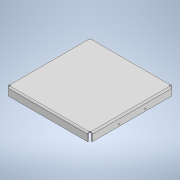
# Autodesk Inventor part: sheetmetaltop2.0
Saved by Autodesk Inventor 2020.2 (Build 242310000, 310)
## iProperties
Created: 2020-02-06
Part Number: sheetmetaltop2.0
Material: Generic
Document SubType Name: Sheet Metal
Designer: ColinP
Density: 1 g/cm^3
Sheet Metal Rule: Default
Appearance: Default
Flat Pattern Width: 27.94 cm
Flat Pattern Length: 27.94 cm
Flat Pattern Area: 780.644 cm^2
Sheet Metal Width: 11.000 in
Sheet Metal Length: 11.000 in
Sheet Metal Area: 121.000 in^2
Author: ColinP
Autodesk Inventor part; units mm, degrees
ref_plane "YZ Plane" through (0, 0, 0) normal (1, 0, 0) x (0, 1, 0)
ref_plane "XZ Plane" through (0, 0, 0) normal (0, 1, 0) x (-1, 0, 0)
ref_plane "XY Plane" through (0, 0, 0) normal (0, 0, 1) x (1, 0, 0)
sketch "Sketch1" plane through (0, 0, 0) normal (0, 1, 0) x (-1, 0, 0)
  line L0 (114.3, 114.3) -> (-114.3, 114.3)
  line L1 (-114.3, 114.3) -> (-114.3, -114.3)
  line L2 (-114.3, -114.3) -> (114.3, -114.3)
  line L3 (114.3, -114.3) -> (114.3, 114.3)
  line L4 (114.3, 114.3) -> (139.7, 114.3)
  line L5 (139.7, 114.3) -> (139.7, -114.3)
  line L6 (139.7, -114.3) -> (114.3, -114.3)
  line L7 (114.3, -114.3) -> (114.3, -139.7)
  line L8 (114.3, -139.7) -> (-114.3, -139.7)
  line L9 (-114.3, -139.7) -> (-114.3, -114.3)
  line L10 (-114.3, -114.3) -> (-139.7, -114.3)
  line L11 (-139.7, -114.3) -> (-139.7, 114.3)
  line L12 (-139.7, 114.3) -> (-114.3, 114.3)
  line L13 (-114.3, 114.3) -> (-114.3, 139.7)
  line L14 (-114.3, 139.7) -> (114.3, 139.7)
  line L15 (114.3, 139.7) -> (114.3, 114.3)
  point P0 (0, 0)
  dimension "d0" = 228.6
  dimension "d1" = 228.6
  dimension "d2" = 25.4
  dimension "d3" = 25.4
  dimension "d4" = 25.4
  dimension "d5" = 25.4
  measures "d0" distance of L2.end L1.end
  measures "d1" distance of L1.end L0.end
  measures "d2" distance of L0.start L4.end
  measures "d3" distance of L2.end L7.end
  measures "d4" distance of L1.end L10.end
  measures "d5" distance of L0.end L13.end
extrude "Plate1" add sketch "Sketch1" along normal blind 3.048
sketch "Sketch3" plane through (0, 0, 0) normal (0, -1, 0) x (1, 0, 0)
  line L0 (-114.3, -114.3) -> (-114.3, -139.7) projected
  line L1 (-114.3, -114.3) -> (-114.3, -116.84)
  line L2 (-114.3, -116.84) -> (114.3, -116.84)
  line L3 (114.3, -139.7) -> (114.3, -114.3) projected
  line L4 (114.3, -116.84) -> (114.3, -114.3)
  point P0 (0, 0)
  dimension "d8" = 2.54
  dimension "d9" = 90
  constraints: 6 end point, 2 point on line
  measures "d8" distance of L0.start L1.end
  measures "d9" angle of L2 L1
fold "Fold1" angle 90 bend radius 1.27 thickness 3.048 k factor 0.44 line from (-114.3, 0, -116.84) to (114.3, 0, -116.84) line at bend start moving side (0, 0, -1) folds toward (0, -1, 0)
sketch "Sketch4" plane through (0, 0, 0) normal (0, -1, 0) x (1, 0, 0)
  line L0 (-139.7, -114.3) -> (-114.3, -114.3) projected
  line L1 (-114.3, -114.3) -> (-116.84, -114.3)
  line L2 (-116.84, -114.3) -> (-116.84, 114.3)
  line L3 (-114.3, 114.3) -> (-139.7, 114.3) projected
  point P0 (0, 0)
  dimension "d16" = 2.54
  constraints: 4 end point, 2 point on line, 1 perpendicular
  measures "d16" distance of L0.end L1.end
fold "Fold2" angle 90 bend radius 1.27 thickness 3.048 k factor 0.44 line from (-116.84, 0, -114.3) to (-116.84, 0, 114.3) line at bend start moving side (-1, 0, 0) folds toward (0, -1, 0)
sketch "Sketch5" plane through (0, 0, 0) normal (0, -1, 0) x (1, 0, 0)
  line L0 (-116.84, 114.3) -> (-114.3, 114.3) projected
  line L1 (-114.3, 114.3) -> (-114.3, 116.84)
  line L2 (-114.3, 114.3) -> (-114.3, 139.7) projected
  line L3 (-114.3, 116.84) -> (114.3, 116.84)
  line L4 (114.3, 139.7) -> (114.3, 114.3) projected
  point P0 (0, 0)
  dimension "d23" = 2.54
  constraints: 4 end point, 2 point on line, 1 perpendicular
  measures "d23" distance of L0.end L1.end
fold "Fold3" angle 90 bend radius 1.27 thickness 3.048 k factor 0.44 line from (-114.3, 0, 116.84) to (114.3, 0, 116.84) line at bend start moving side (0, 0, 1) folds toward (0, -1, 0)
sketch "Sketch6" plane through (0, 0, 0) normal (0, -1, 0) x (1, 0, 0)
  line L0 (114.3, -116.84) -> (114.3, -114.3) projected
  line L1 (114.3, -114.3) -> (116.84, -114.3)
  line L2 (114.3, -114.3) -> (139.7, -114.3) projected
  line L3 (116.84, -114.3) -> (116.84, 114.3)
  line L4 (139.7, 114.3) -> (114.3, 114.3) projected
  point P0 (0, 0)
  dimension "d30" = 2.54
  constraints: 4 end point, 2 point on line, 1 perpendicular
  measures "d30" distance of L0.end L1.end
fold "Fold4" angle 90 bend radius 1.27 thickness 3.048 k factor 0.44 line from (116.84, 0, -114.3) to (116.84, 0, 114.3) line at bend start moving side (1, 0, 0) folds toward (0, -1, 0)
sketch "Sketch7" plane through (-121.158, -20.0285, -114.3) normal (-1, 0, 0) x (0, 0, 1)
  line L0 (0, 18.7585) -> (228.6, 18.7585) projected
  line L1 (0, 18.7585) -> (0, 6.0585)
  line L2 (0, 0) -> (0, 18.7585) projected
  line L3 (0, 6.0585) -> (76.2, 6.0585)
  line L4 (76.2, 6.0585) -> (152.4, 6.0585)
  point P0 (114.3, 20.0285)
  dimension "d37" = 12.7
  dimension "d38" = 76.2
  dimension "d39" = 76.2
  constraints: 6 end point, 2 point on line, 1 horizontal
  measures "d37" distance of L0.start L1.end
  measures "d38" distance of L1.end L3.end
  measures "d39" distance of L3.end L4.end
hole "Hole1" at (-121.158, -13.97, 38.1) at (-121.158, -13.97, -38.1) direction (1, 0, 0) diameter 3.2766 end through all clearance for "Flat Head Machine Screw (82)" size "#4" standard "Ansi Unified Screw Threads"
equation "\"d6\" = Thickness"
equation "\"d10\" = BendReliefWidth"
equation "\"d11\" = BendReliefDepth"
equation "\"d12\" = MinimumRemnant"
equation "\"d13\" = TransitionRadius"
equation "\"d17\" = BendReliefWidth"
equation "\"d18\" = BendReliefDepth"
equation "\"d19\" = MinimumRemnant"
equation "\"d20\" = TransitionRadius"
equation "\"d24\" = BendReliefWidth"
equation "\"d25\" = BendReliefDepth"
equation "\"d26\" = MinimumRemnant"
equation "\"d27\" = TransitionRadius"
equation "\"d31\" = BendReliefWidth"
equation "\"d32\" = BendReliefDepth"
equation "\"d33\" = MinimumRemnant"
equation "\"d34\" = TransitionRadius"
equation "\"d45\" = Thickness"
equation "\"BendRadius\" = Thickness"
equation "\"BendReliefWidth\" = Thickness"
equation "\"BendReliefDepth\" = 0.5 * Thickness"
equation "\"CornerReliefSize\" = 4 * Thickness"
equation "\"MinimumRemnant\" = 2 * Thickness"
equation "\"TransitionRadius\" = BendRadius"
equation "\"JacobiRadiusSize\" = BendRadius"
equation "\"GapSize\" = Thickness"
equation "\"Thickness\" = 3.048"
body "Solid1"
